Autodesk Inventor part; units mm, degrees
(part 2 of 2)
  line L197 (11.6356, -9.684) -> (11.6356, -8.9363) construction
  line L198 (11.6356, -8.9363) -> (11.5503, -8.9363) construction
  line L199 (11.5503, -8.9363) -> (11.5503, -9.8863) construction
  line L200 (11.5503, -9.8863) -> (11.5697, -9.8863) construction
  line L201 (11.5697, -9.8863) -> (12.1958, -9.1403) construction
  line L202 (12.1958, -9.1403) -> (12.1958, -9.8863) construction
  spline S63 degree 3 poles (12.9637, -8.912) (12.9539, -8.9121) (12.9344, -8.9124) (12.9054, -8.9146) (12.8768, -8.918) (12.8486, -8.9227) (12.8209, -8.9291) (12.7937, -8.9367) (12.7668, -8.9456) (12.7405, -8.9562) (12.7144, -8.9682) (12.6884, -8.9817) (12.6627, -8.9969) (12.6371, -9.014) (12.6116, -9.0325) (12.5866, -9.0531) (12.5613, -9.0749) (12.5451, -9.0905) (12.5369, -9.0985) knots 0 0 0 0 0.061617 0.122179 0.182216 0.241864 0.30096 0.359969 0.419033 0.478069 0.537993 0.59896 0.661321 0.725248 0.79122 0.858746 0.928318 1 1 1 1 construction
  line L203 (12.5369, -9.0985) -> (12.6099, -9.1677) construction
  spline S64 degree 3 poles (12.6099, -9.1677) (12.6232, -9.1553) (12.6493, -9.1307) (12.6919, -9.0988) (12.7363, -9.0715) (12.7824, -9.0493) (12.829, -9.0315) (12.8753, -9.0189) (12.9211, -9.0108) (12.9516, -9.0099) (12.9666, -9.0094) knots 0 0 0 0 0.136144 0.269043 0.398517 0.5271 0.652283 0.77168 0.887495 1 1 1 1 construction
  spline S65 degree 3 poles (12.9666, -9.0094) (12.9758, -9.0095) (12.9942, -9.0097) (13.0215, -9.0126) (13.0485, -9.0167) (13.0752, -9.0227) (13.1016, -9.0302) (13.1276, -9.0397) (13.1533, -9.0507) (13.1784, -9.0634) (13.2028, -9.0774) (13.2258, -9.0929) (13.2476, -9.1094) (13.2678, -9.1273) (13.2865, -9.1465) (13.3041, -9.1666) (13.32, -9.1881) (13.3345, -9.2108) (13.3473, -9.234) (13.3587, -9.2578) (13.3682, -9.2819) (13.3757, -9.3063) (13.3819, -9.331) (13.3863, -9.3561) (13.3888, -9.3815) (13.3892, -9.3986) (13.3894, -9.4071) knots 0 0 0 0 0.042841 0.085571 0.127719 0.170068 0.212787 0.255482 0.298877 0.342861 0.386528 0.429532 0.471886 0.513729 0.555082 0.596535 0.63812 0.679822 0.721331 0.761888 0.802199 0.841806 0.88106 0.920633 0.960101 1 1 1 1 construction
  spline S66 degree 3 poles (13.3894, -9.4071) (13.3892, -9.4159) (13.3888, -9.4334) (13.3862, -9.4595) (13.3813, -9.4852) (13.3748, -9.5107) (13.3667, -9.5358) (13.3565, -9.5606) (13.3445, -9.585) (13.3306, -9.6089) (13.3154, -9.6321) (13.2983, -9.6539) (13.2801, -9.6747) (13.2603, -9.694) (13.2393, -9.7123) (13.2166, -9.7291) (13.1927, -9.7447) (13.1674, -9.7589) (13.1412, -9.7716) (13.1142, -9.7829) (13.0865, -9.7922) (13.0582, -9.7998) (13.0294, -9.806) (12.9998, -9.81) (12.9697, -9.8129) (12.9494, -9.8131) (12.9392, -9.8133) knots 0 0 0 0 0.038994 0.077882 0.116652 0.155416 0.194618 0.234261 0.274547 0.315667 0.35702 0.398083 0.439098 0.479833 0.521274 0.562841 0.605292 0.648409 0.691727 0.735149 0.778369 0.821661 0.865524 0.909731 0.954523 1 1 1 1 construction
  spline S67 degree 3 poles (12.9392, -9.8133) (12.9268, -9.813) (12.9027, -9.8125) (12.8671, -9.8086) (12.833, -9.8024) (12.8003, -9.7934) (12.7691, -9.7819) (12.7393, -9.7681) (12.7111, -9.7514) (12.6843, -9.7325) (12.6597, -9.7114) (12.6375, -9.6887) (12.618, -9.6645) (12.6011, -9.6388) (12.587, -9.6115) (12.5755, -9.5827) (12.5667, -9.5524) (12.5631, -9.5315) (12.5612, -9.5209) knots 0 0 0 0 0.07063 0.138694 0.204918 0.269441 0.332636 0.395302 0.457764 0.520657 0.582852 0.643315 0.70258 0.760908 0.81949 0.878269 0.938491 1 1 1 1 construction
  line L204 (12.5612, -9.5209) -> (12.8779, -9.5209) construction
  line L205 (12.8779, -9.5209) -> (12.8779, -9.4235) construction
  line L206 (12.8779, -9.4235) -> (12.476, -9.4235) construction
  spline S68 degree 3 poles (12.476, -9.4235) (12.4764, -9.4417) (12.4773, -9.4772) (12.4837, -9.5291) (12.494, -9.578) (12.508, -9.6241) (12.5261, -9.6674) (12.5482, -9.7078) (12.5746, -9.7451) (12.6043, -9.7796) (12.6377, -9.8103) (12.6738, -9.8373) (12.7126, -9.8601) (12.7543, -9.8787) (12.7985, -9.8931) (12.8455, -9.9034) (12.8952, -9.9095) (12.9292, -9.9103) (12.9466, -9.9107) knots 0 0 0 0 0.071272 0.139493 0.204635 0.267406 0.328446 0.388397 0.447734 0.507392 0.566768 0.625478 0.684067 0.743248 0.804033 0.866499 0.931723 1 1 1 1 construction
  spline S69 degree 3 poles (12.9466, -9.9107) (12.9573, -9.9105) (12.9785, -9.9102) (13.0097, -9.9081) (13.0401, -9.9047) (13.0696, -9.8997) (13.0983, -9.8935) (13.1262, -9.8856) (13.1533, -9.8765) (13.1796, -9.8661) (13.2049, -9.8541) (13.2293, -9.8407) (13.253, -9.826) (13.2758, -9.8098) (13.2978, -9.7923) (13.3189, -9.7732) (13.3391, -9.7528) (13.3518, -9.7383) (13.3582, -9.731) knots 0 0 0 0 0.069237 0.136557 0.202094 0.266464 0.329769 0.391879 0.453271 0.514115 0.57439 0.634142 0.693923 0.754152 0.81447 0.875661 0.937348 1 1 1 1 construction
  spline S70 degree 3 poles (13.3582, -9.731) (13.3675, -9.7195) (13.3859, -9.6965) (13.4096, -9.6597) (13.4298, -9.6216) (13.4462, -9.5821) (13.459, -9.5412) (13.4681, -9.499) (13.4735, -9.4554) (13.4743, -9.4259) (13.4747, -9.411) knots 0 0 0 0 0.127896 0.253668 0.376738 0.499344 0.621999 0.745699 0.871345 1 1 1 1 construction
  spline S71 degree 3 poles (13.4747, -9.411) (13.4745, -9.3998) (13.4743, -9.3776) (13.4708, -9.3446) (13.4658, -9.3122) (13.4584, -9.2805) (13.4492, -9.2493) (13.4376, -9.2187) (13.4242, -9.1886) (13.4086, -9.1593) (13.3912, -9.1312) (13.3723, -9.1044) (13.3516, -9.0793) (13.3296, -9.0556) (13.3059, -9.0337) (13.2807, -9.0133) (13.2541, -8.9944) (13.2258, -8.9773) (13.1965, -8.9619) (13.1661, -8.9485) (13.1346, -8.9373) (13.1023, -8.9279) (13.0689, -8.9209) (13.0348, -8.9159) (12.9996, -8.9124) (12.9758, -8.9121) (12.9637, -8.912) knots 0 0 0 0 0.042039 0.083544 0.124643 0.165303 0.206171 0.246971 0.288329 0.329987 0.371797 0.412738 0.453459 0.494001 0.534381 0.574952 0.615892 0.65725 0.699007 0.740486 0.782325 0.824567 0.867041 0.9105 0.954619 1 1 1 1 construction
  line L207 (47.1288, -8.7194) -> (47.1288, -7.7194) construction
  line L208 (47.1288, -7.7194) -> (46.9026, -7.7194) construction
  spline S72 degree 3 poles (46.9026, -7.7194) (46.885, -7.7196) (46.8509, -7.7198) (46.8015, -7.7225) (46.7556, -7.7266) (46.7131, -7.7323) (46.6742, -7.7398) (46.6388, -7.7492) (46.6068, -7.7601) (46.578, -7.7729) (46.5517, -7.7879) (46.5267, -7.8045) (46.5031, -7.8234) (46.4805, -7.8443) (46.4593, -7.8675) (46.439, -7.8927) (46.4202, -7.9201) (46.4024, -7.9492) (46.3862, -7.9801) (46.3721, -8.0125) (46.3603, -8.0462) (46.3507, -8.0812) (46.3431, -8.1175) (46.3377, -8.155) (46.3344, -8.1938) (46.3341, -8.2201) (46.3339, -8.2335) knots 0 0 0 0 0.060148 0.116267 0.168654 0.217399 0.262434 0.303933 0.34226 0.377441 0.411406 0.445398 0.479766 0.514584 0.550214 0.587001 0.624663 0.663615 0.703456 0.74345 0.784013 0.825133 0.867265 0.910306 0.954424 1 1 1 1 construction
  spline S73 degree 3 poles (46.3339, -8.2335) (46.3344, -8.2523) (46.3353, -8.2894) (46.3427, -8.3439) (46.3546, -8.3961) (46.3715, -8.4457) (46.3923, -8.4921) (46.4172, -8.5346) (46.4459, -8.573) (46.4778, -8.607) (46.5125, -8.6363) (46.5485, -8.6613) (46.5861, -8.6811) (46.6194, -8.6936) (46.6482, -8.7014) (46.6734, -8.706) (46.7022, -8.7102) (46.7346, -8.7135) (46.7706, -8.7164) (46.8103, -8.7179) (46.8536, -8.7193) (46.8836, -8.7194) (46.8992, -8.7194) knots 0 0 0 0 0.065773 0.129478 0.19143 0.252446 0.311787 0.368818 0.424092 0.478492 0.531394 0.582004 0.631201 0.679503 0.705561 0.735222 0.769132 0.806858 0.84893 0.895117 0.94547 1 1 1 1 construction
  line L209 (46.8992, -8.7194) -> (47.1288, -8.7194) construction
  line L210 (47.8467, -8.7194) -> (47.8467, -7.7194) construction
  line L211 (47.8467, -7.7194) -> (47.3083, -7.7194) construction
  line L212 (47.3083, -7.7194) -> (47.3083, -7.8989) construction
  line L213 (47.3083, -7.8989) -> (47.6673, -7.8989) construction
  line L214 (47.6673, -7.8989) -> (47.6673, -8.0912) construction
  line L215 (47.6673, -8.0912) -> (47.3083, -8.0912) construction
  line L216 (47.3083, -8.0912) -> (47.3083, -8.2707) construction
  line L217 (47.3083, -8.2707) -> (47.6673, -8.2707) construction
  line L218 (47.6673, -8.2707) -> (47.6673, -8.54) construction
  line L219 (47.6673, -8.54) -> (47.3083, -8.54) construction
  line L220 (47.3083, -8.54) -> (47.3083, -8.7194) construction
  line L221 (47.3083, -8.7194) -> (47.8467, -8.7194) construction
  line L222 (48.4621, -8.7194) -> (48.4621, -7.7194) construction
  line L223 (48.4621, -7.7194) -> (48.2826, -7.7194) construction
  line L224 (48.2826, -7.7194) -> (48.2826, -8.54) construction
  line L225 (48.2826, -8.54) -> (48.0006, -8.54) construction
  line L226 (48.0006, -8.54) -> (48.0006, -8.7194) construction
  line L227 (48.0006, -8.7194) -> (48.4621, -8.7194) construction
  circle A18 centre (48.35, -12.79) radius 0.75 construction
  circle A19 centre (48.35, -10.25) radius 0.75 construction
  circle A20 centre (9.37, -17.12) radius 0.75 construction
  circle A21 centre (9.37, -14.58) radius 0.75 construction
  circle A22 centre (9.37, -12.04) radius 0.75 construction
  circle A23 centre (9.37, -9.5) radius 0.75 construction
  line L228 (25.55, -16.65) -> (24.65, -16.65) construction
  line L229 (25.55, -15.85) -> (25.55, -16.65) construction
  line L230 (24.65, -15.85) -> (25.55, -15.85) construction
  line L231 (24.65, -16.65) -> (24.65, -15.85) construction
  line L232 (25.55, -15.35) -> (24.65, -15.35) construction
  line L233 (25.55, -14.55) -> (25.55, -15.35) construction
  line L234 (24.65, -14.55) -> (25.55, -14.55) construction
  line L235 (24.65, -15.35) -> (24.65, -14.55) construction
  line L236 (25.55, -14.05) -> (24.65, -14.05) construction
  line L237 (25.55, -13.25) -> (25.55, -14.05) construction
  line L238 (24.65, -13.25) -> (25.55, -13.25) construction
  line L239 (24.65, -14.05) -> (24.65, -13.25) construction
  line L240 (25.55, -12.75) -> (24.65, -12.75) construction
  line L241 (25.55, -11.95) -> (25.55, -12.75) construction
  line L242 (24.65, -11.95) -> (25.55, -11.95) construction
  line L243 (24.65, -12.75) -> (24.65, -11.95) construction
  line L244 (25.55, -11.45) -> (24.65, -11.45) construction
  line L245 (25.55, -10.65) -> (25.55, -11.45) construction
  line L246 (24.65, -10.65) -> (25.55, -10.65) construction
  line L247 (24.65, -11.45) -> (24.65, -10.65) construction
  line L248 (25.55, -10.15) -> (24.65, -10.15) construction
  line L249 (25.55, -9.35) -> (25.55, -10.15) construction
  line L250 (24.65, -9.35) -> (25.55, -9.35) construction
  line L251 (24.65, -10.15) -> (24.65, -9.35) construction
  line L252 (25.55, -8.85) -> (24.65, -8.85) construction
  line L253 (25.55, -8.05) -> (25.55, -8.85) construction
  line L254 (24.65, -8.05) -> (25.55, -8.05) construction
  line L255 (24.65, -8.85) -> (24.65, -8.05) construction
  line L256 (25.55, -17.15) -> (25.55, -17.95) construction
  line L257 (24.65, -17.15) -> (25.55, -17.15) construction
  line L258 (24.65, -17.95) -> (24.65, -17.15) construction
  line L259 (25.55, -17.95) -> (24.65, -17.95) construction
  line L260 (26.5, -7.75) -> (33.8, -7.75) construction
  line L261 (26.5, -18.25) -> (26.5, -7.75) construction
  line L262 (33.8, -18.25) -> (26.5, -18.25) construction
  line L263 (33.8, -7.75) -> (33.8, -18.25) construction
  line L264 (34.75, -8.05) -> (35.65, -8.05) construction
  line L265 (34.75, -8.05) -> (34.75, -8.85) construction
  line L266 (35.65, -8.85) -> (34.75, -8.85) construction
  line L267 (35.65, -8.05) -> (35.65, -8.85) construction
  line L268 (34.75, -9.35) -> (35.65, -9.35) construction
  line L269 (34.75, -9.35) -> (34.75, -10.15) construction
  line L270 (35.65, -10.15) -> (34.75, -10.15) construction
  line L271 (35.65, -9.35) -> (35.65, -10.15) construction
  line L272 (34.75, -10.65) -> (35.65, -10.65) construction
  line L273 (34.75, -10.65) -> (34.75, -11.45) construction
  line L274 (35.65, -11.45) -> (34.75, -11.45) construction
  line L275 (35.65, -10.65) -> (35.65, -11.45) construction
  line L276 (34.75, -11.95) -> (35.65, -11.95) construction
  line L277 (34.75, -11.95) -> (34.75, -12.75) construction
  line L278 (35.65, -12.75) -> (34.75, -12.75) construction
  line L279 (35.65, -11.95) -> (35.65, -12.75) construction
  line L280 (34.75, -13.25) -> (35.65, -13.25) construction
  line L281 (34.75, -13.25) -> (34.75, -14.05) construction
  line L282 (35.65, -14.05) -> (34.75, -14.05) construction
  line L283 (35.65, -13.25) -> (35.65, -14.05) construction
  line L284 (34.75, -14.55) -> (35.65, -14.55) construction
  line L285 (34.75, -14.55) -> (34.75, -15.35) construction
  line L286 (35.65, -15.35) -> (34.75, -15.35) construction
  line L287 (35.65, -14.55) -> (35.65, -15.35) construction
  line L288 (34.75, -15.85) -> (35.65, -15.85) construction
  line L289 (34.75, -15.85) -> (34.75, -16.65) construction
  line L290 (35.65, -16.65) -> (34.75, -16.65) construction
  line L291 (35.65, -15.85) -> (35.65, -16.65) construction
  line L292 (34.75, -17.15) -> (35.65, -17.15) construction
  line L293 (34.75, -17.15) -> (34.75, -17.95) construction
  line L294 (35.65, -17.95) -> (34.75, -17.95) construction
  line L295 (35.65, -17.15) -> (35.65, -17.95) construction
  circle A24 centre (45.56, -5.5) radius 0.75 construction
  circle A25 centre (48.1, -5.5) radius 0.75 construction
  line L296 (50.7939, -3) -> (5.9071, -3) construction
  line L297 (5.9071, -3) -> (5.9071, -23.644) construction
  line L298 (5.9071, -23.644) -> (50.7939, -23.644) construction
  line L299 (50.7939, -23.644) -> (50.7939, -3) construction
  line L300 (50.7939, -23.644) -> (5.9071, -23.644)
  line L301 (5.9071, -23.644) -> (5.9071, -3)
  line L302 (5.9071, -3) -> (50.7939, -3)
  line L303 (50.7939, -3) -> (50.7939, -23.644)
  line L304 (93.3881, -56.8601) -> (4, -56.8601)
  line L305 (4, -56.8601) -> (4, -8.85)
  line L306 (4, -8.85) -> (93.3881, -8.85)
  line L307 (93.3881, -8.85) -> (93.3881, -56.8601)
  point P0 (0, -3)
  constraints: 24 end point, 6 parallel, 3 horizontal, 3 perpendicular
extrude "Extrusion5" cut sketch "Sketch5" against normal blind 3
sketch "Sketch6" plane through (103, 6.6, 3) normal (1, 0, 0) x (0, 0, -1)
  line L0 (32.7723, 17.3458) -> (40.0033, 0.6221) projected
  arc A0 (33.8143, 19.9753) -> (32.7723, 17.3458) centre (34.6081, 18.1395) ccw projected
  line L1 (49.8404, 26.9047) -> (33.8143, 19.9753) projected
  arc A1 (52.4699, 25.8626) -> (49.8404, 26.9047) centre (50.6341, 25.0689) ccw projected
  line L2 (59.7009, 9.139) -> (52.4699, 25.8626) projected
  arc A2 (58.6589, 6.5095) -> (59.7009, 9.139) centre (57.8651, 8.3452) ccw projected
  line L3 (42.6328, -0.4199) -> (58.6589, 6.5095) projected
  arc A3 (40.0033, 0.6221) -> (42.6328, -0.4199) centre (41.8391, 1.4159) ccw projected
  arc A4 (58.778, 6.2341) -> (59.9763, 9.2581) centre (57.8651, 8.3452) ccw
  line L4 (59.9763, 9.2581) -> (52.7452, 25.9817)
  arc A5 (52.7452, 25.9817) -> (49.7213, 27.18) centre (50.6341, 25.0689) ccw
  line L5 (49.7213, 27.18) -> (33.6952, 20.2506)
  arc A6 (33.6952, 20.2506) -> (32.4969, 17.2267) centre (34.6081, 18.1395) ccw
  line L6 (32.4969, 17.2267) -> (39.728, 0.503)
  arc A7 (39.728, 0.503) -> (42.7519, -0.6953) centre (41.8391, 1.4159) ccw
  line L7 (42.7519, -0.6953) -> (58.778, 6.2341)
  point P0 (3, -6.6)
  dimension "d16" = 0.3
  constraints: 8 end point, 8 point on circle, 4 centre point, 7 other
  measures "d16" distance between parallel lines of L3 L7
extrude "Extrusion6" cut sketch "Sketch6" against normal through all contours A0 L1 A1 L2 A2 L3 A3 L0 | L7 A7 L6 A6 L5 A5 L4 A4
sketch "Sketch7" plane through (-2, 6.6, 0) normal (1, 0, 0) x (0, 0, -1)
  arc A0 (36.728, 0.503) -> (37.0265, 0) centre (38.8391, 1.4159) ccw projected
  line L0 (36.728, 0.503) -> (29.4969, 17.2267) projected
  arc A1 (30.6952, 20.2506) -> (29.4969, 17.2267) centre (31.6081, 18.1395) ccw projected
  line L1 (30.6952, 20.2506) -> (46.7213, 27.18) projected
  arc A2 (49.7452, 25.9817) -> (46.7213, 27.18) centre (47.6341, 25.0689) ccw projected
  line L2 (49.7452, 25.9817) -> (56.9763, 9.2581) projected
  arc A3 (55.778, 6.2341) -> (56.9763, 9.2581) centre (54.8651, 8.3452) ccw projected
  line L3 (55.778, 6.2341) -> (41.3598, 0) projected
  line L4 (41.3598, 0) -> (60, 0) projected
  line L5 (60, 0) -> (60, 4.0286) projected
  line L6 (60, 4.0286) -> (27.1513, 80) projected
  line L7 (-3, 80) -> (27.1513, 80) projected
  line L8 (-3, 0) -> (-3, 80) projected
  line L9 (-3, 0) -> (37.0265, 0) projected
  circle A4 centre (17.557, 24.8509) radius 11.8979 projected
  line L10 (45.542, 26.6701) -> (30.6952, 20.2506)
  line L11 (30.6952, 20.2506) -> (29.5936, 22.7985)
  line L12 (29.5936, 22.7985) -> (44.4403, 29.218)
  line L13 (44.4403, 29.218) -> (45.542, 26.6701)
  line L14 (29.4969, 17.2267) -> (37.0265, 0)
  line L15 (37.0265, 0) -> (33.9632, -1.339)
  line L16 (33.9632, -1.339) -> (26.4336, 15.8878)
  line L17 (26.4336, 15.8878) -> (29.4969, 17.2267)
  line L18 (54.8651, 5.8395) -> (41.3598, 0)
  line L19 (57.4122, -0.0512) -> (54.8651, 5.8395)
  line L20 (29.5936, 22.7985) -> (29.2312, 22.5542)
  line L21 (26.4336, 15.8878) -> (26.1097, 16.5797)
  line L22 (44.4403, 29.218) -> (48.3733, 30.9185)
  line L23 (33.9632, -1.339) -> (35.3257, -4.4564)
  line L24 (35.3257, -4.4564) -> (60, -4.4564)
  line L25 (41.3598, 0) -> (60, 0) projected
  line L26 (60, -4.4564) -> (60, 4.0286)
  point P0 (0, -6.6)
  constraints: 32 end point, 5 parallel, 5 point on line, 3 perpendicular, 2 point on circle, 1 collinear, 2 other
extrude "Extrusion7" add sketch "Sketch7" along normal blind 15 contours L0 L14 A0 | A0 L9 L16 L17 L0 | L15 L16 L9 | L14 A1 L1 A2 L2 A3 L3 L4 L26 L24 L23 L15 | L17 L21 A4 L20 L11 A1 | L11 L12 L13 L1 | L13 L22 L6 L5 L4 L19 L3 A3 L2 A2 L1 | A4 | L4 L3 L19
sketch "Sketch8" plane through (-5, 6.6, 3) normal (-1, 0, 0) x (0, 0, 1)
  line L0 (-42.7519, -0.6953) -> (-58.778, 6.2341) projected
  arc A0 (-42.7519, -0.6953) -> (-39.728, 0.503) centre (-41.8391, 1.4159) ccw projected
  line L1 (-39.728, 0.503) -> (-32.4969, 17.2267) projected
  arc A1 (-32.4969, 17.2267) -> (-33.6952, 20.2506) centre (-34.6081, 18.1395) ccw projected
  line L2 (-33.6952, 20.2506) -> (-49.7213, 27.18) projected
  arc A2 (-49.7213, 27.18) -> (-52.7452, 25.9817) centre (-50.6341, 25.0689) ccw projected
  line L3 (-52.7452, 25.9817) -> (-59.9763, 9.2581) projected
  arc A3 (-59.9763, 9.2581) -> (-58.778, 6.2341) centre (-57.8651, 8.3452) ccw projected
  circle A4 centre (-20.557, 24.8509) radius 10.6399 projected
  circle A5 centre (-20.557, 24.8509) radius 11.9384
  point P0 (-3, -6.6)
  constraints: 1 centre point
extrude "Extrusion8" cut sketch "Sketch8" against normal through all contours L0 A3 L3 A2 L2 A1 L1 A0 | A4 | A5
sketch "Sketch9" plane through (100, 6.6, 0) normal (-1, 0, 0) x (0, 0, 1)
  arc A0 (-29.2786, 22.5862) -> (-26.1281, 16.5405) centre (-17.557, 24.8509) ccw projected
  line L0 (-53.8601, -2) -> (-53.8601, -4.4564) projected
  line L1 (-60, -2) -> (-53.8601, -2) projected
  line L2 (-60, -2) -> (-60, 4.0286) projected
  line L3 (-60, 4.0286) -> (-48.3733, 30.9185) projected
  line L4 (-48.3733, 30.9185) -> (-29.5936, 22.7985) projected
  line L5 (-29.5936, 22.7985) -> (-29.2786, 22.5862) projected
  line L6 (-26.1281, 16.5405) -> (-26.4336, 15.8878) projected
  line L7 (-26.4336, 15.8878) -> (-35.3257, -4.4564) projected
  line L8 (-35.3257, -4.4564) -> (-53.8601, -4.4564) projected
  line L9 (-41.5802, 6.1987) -> (-40.8052, 7.9911) projected
  line L10 (-40.8052, 7.9911) -> (-48.7279, 11.4167) projected
  line L11 (-48.7279, 11.4167) -> (-49.5029, 9.6243) projected
  line L12 (-49.5029, 9.6243) -> (-41.5802, 6.1987) projected
  line L13 (-36.158, 12.8961) -> (-34.2689, 17.2651) projected
  line L14 (-34.2689, 17.2651) -> (-46.4486, 22.5313) projected
  line L15 (-46.4486, 22.5313) -> (-48.3377, 18.1624) projected
  line L16 (-48.3377, 18.1624) -> (-36.158, 12.8961) projected
  line L17 (-29.7723, 17.3458) -> (-37.0033, 0.6221) projected
  arc A1 (-39.6328, -0.4199) -> (-37.0033, 0.6221) centre (-38.8391, 1.4159) ccw projected
  line L18 (-39.6328, -0.4199) -> (-55.6589, 6.5095) projected
  arc A2 (-56.7009, 9.139) -> (-55.6589, 6.5095) centre (-54.8651, 8.3452) ccw projected
  line L19 (-56.7009, 9.139) -> (-49.4699, 25.8626) projected
  arc A3 (-46.8404, 26.9047) -> (-49.4699, 25.8626) centre (-47.6341, 25.0689) ccw projected
  line L20 (-46.8404, 26.9047) -> (-30.8143, 19.9753) projected
  arc A4 (-29.7723, 17.3458) -> (-30.8143, 19.9753) centre (-31.6081, 18.1395) ccw projected
  line L21 (-36.8772, 0.5676) -> (-29.6462, 17.2912)
  arc A5 (-29.6462, 17.2912) -> (-30.7598, 20.1014) centre (-31.6081, 18.1395) ccw
  line L22 (-30.7598, 20.1014) -> (-46.7859, 27.0308)
  arc A6 (-46.7859, 27.0308) -> (-49.596, 25.9172) centre (-47.6341, 25.0689) ccw
  line L23 (-49.596, 25.9172) -> (-56.827, 9.1935)
  arc A7 (-56.827, 9.1935) -> (-55.7134, 6.3834) centre (-54.8651, 8.3452) ccw
  line L24 (-55.7134, 6.3834) -> (-39.6873, -0.546)
  arc A8 (-39.6873, -0.546) -> (-36.8772, 0.5676) centre (-38.8391, 1.4159) ccw
  point P0 (0, -6.6)
  constraints: 8 end point, 8 point on circle, 4 centre point, 7 other
extrude "Extrusion9" add sketch "Sketch9" along normal blind 10 contours A0 L6 L7 L8 L0 L1 L2 L3 L4 L5 | A8 L24 A7 L23 A6 L22 A5 L21
sketch "Sketch10" plane through (0, 0, 0) normal (0, 0, -1) x (-1, 0, 0)
  line L0 (5, 10.6286) -> (-13, 10.6286) projected
  line L1 (5, 86.6) -> (5, 10.6286) projected
  arc A0 (5, 86.6) -> (0, 91.6) centre (0, 86.6) ccw projected
  line L2 (-98, 91.6) -> (0, 91.6) projected
  arc A1 (-98, 91.6) -> (-103, 86.6) centre (-98, 86.6) ccw projected
  line L3 (-103, 10.6286) -> (-103, 86.6) projected
  line L4 (-90, 10.6286) -> (-103, 10.6286) projected
  line L5 (-90, 37.5185) -> (-90, 10.6286) projected
  line L6 (-100, 37.5185) -> (-90, 37.5185) projected
  line L7 (-100, 86.6) -> (-100, 37.5185) projected
  arc A2 (-98, 88.6) -> (-100, 86.6) centre (-98, 86.6) ccw projected
  line L8 (0, 88.6) -> (-98, 88.6) projected
  arc A3 (2, 86.6) -> (0, 88.6) centre (0, 86.6) ccw projected
  line L9 (2, 37.5185) -> (2, 86.6) projected
  line L10 (2, 37.5185) -> (-13, 37.5185) projected
  line L11 (-13, 10.6286) -> (-13, 37.5185) projected
  circle A4 centre (0, 86.6) radius 2 construction
  circle A5 centre (0, 86.6) radius 5
  circle A6 centre (-98, 86.6) radius 2 construction
  circle A7 centre (-98, 86.6) radius 5
  circle A8 centre (0, 86.6) radius 1.45
  circle A9 centre (-98, 86.6) radius 1.45
  point P0 (0, 0)
  dimension "d27" = 2.9
  dimension "d28" = 2.9
  constraints: 6 centre point, 6 coincident, 3 concentric
  measures "d27" diameter of A8
  measures "d28" diameter of A9
extrude "Extrusion10" add sketch "Sketch10" along normal up to surface contours A5 L9 A3 L8 A0 | A5 L8 A3 L9 | A7 L8 A2 L7 A1 | A7 L7 A2 L8 surface through (-5, 93.7327, -24.0673) normal (0, -0.3968725, 0.9178738)
sketch "Sketch11" plane through (98, 1.6, -60) normal (0, 0, -1) x (-1, 0, 0)
  line L0 (8, 9.0286) -> (-5, 9.0286) projected
  line L1 (-5, 5) -> (-5, 9.0286) projected
  arc A0 (-5, 5) -> (0, 0) centre (0, 5) ccw projected
  line L2 (98, 0) -> (0, 0) projected
  arc A1 (98, 0) -> (103, 5) centre (98, 5) ccw projected
  line L3 (103, 9.0286) -> (103, 5) projected
  line L4 (103, 9.0286) -> (85, 9.0286) projected
  line L5 (85, 3) -> (85, 9.0286) projected
  line L6 (8, 3) -> (85, 3) projected
  line L7 (8, 9.0286) -> (8, 3) projected
  circle A2 centre (98, 5) radius 1.45
  circle A3 centre (0, 5) radius 1.45
  point P0 (98, -1.6)
  dimension "d29" = 2.9
  dimension "d30" = 2.9
  constraints: 2 centre point, 2 coincident
  measures "d29" diameter of A2
  measures "d30" diameter of A3
extrude "Extrusion11" cut sketch "Sketch11" against normal blind 20 contours A2 | A3
sketch "Sketch12" plane through (4, 2.1436, -53.8601) normal (0, -1, 0) x (1, 0, 0)
  circle A0 centre (-1.5, -3.6399) radius 1.5 projected
  circle A1 centre (91.5, -3.6399) radius 1.5 projected
  point P0 (-4, 53.8601)
extrude "Extrusion12" cut sketch "Sketch12" against normal blind 20
sketch "Sketch13" plane through (103, 6.6, 3) normal (1, 0, 0) x (0, 0, -1)
  circle A0 centre (20.557, 24.8509) radius 11.9384 projected
  arc A1 (39.728, 0.503) -> (40.0265, 0) centre (41.8391, 1.4159) ccw projected
  line L0 (39.728, 0.503) -> (32.4969, 17.2267) projected
  arc A2 (33.6952, 20.2506) -> (32.4969, 17.2267) centre (34.6081, 18.1395) ccw projected
  line L1 (33.6952, 20.2506) -> (49.7213, 27.18) projected
  arc A3 (52.7452, 25.9817) -> (49.7213, 27.18) centre (50.6341, 25.0689) ccw projected
  line L2 (52.7452, 25.9817) -> (59.9763, 9.2581) projected
  arc A4 (58.778, 6.2341) -> (59.9763, 9.2581) centre (57.8651, 8.3452) ccw projected
  line L3 (58.778, 6.2341) -> (44.3598, 0) projected
  line L4 (44.3598, 0) -> (63, 0) projected
  line L5 (63, 0) -> (63, 4.0286) projected
  line L6 (63, 4.0286) -> (30.1513, 80) projected
  line L7 (0, 80) -> (30.1513, 80) projected
  line L8 (0, 0) -> (0, 80) projected
  line L9 (0, 0) -> (40.0265, 0) projected
  line L10 (3, 75.4174) -> (32.1327, 75.4174) projected
  line L11 (9.8433, 61.5372) -> (8.9292, 61.5372)
  line L12 (5.9292, 64.5372) -> (5.9292, 72.4174)
  line L13 (8.9292, 75.4174) -> (9.8433, 75.4174)
  line L14 (12.8433, 72.4174) -> (12.8433, 64.5372)
  arc A5 (9.8433, 61.5372) -> (12.8433, 64.5372) centre (9.8433, 64.5372) ccw
  arc A6 (5.9292, 64.5372) -> (8.9292, 61.5372) centre (8.9292, 64.5372) ccw
  arc A7 (8.9292, 75.4174) -> (5.9292, 72.4174) centre (8.9292, 72.4174) ccw
  arc A8 (12.8433, 72.4174) -> (9.8433, 75.4174) centre (9.8433, 72.4174) ccw
  point P0 (3, -6.6)
  point P1 (5.9292, 75.4174)
  dimension "d35" = 3
  constraints: 8 end point, 8 point on circle, 8 tangent, 4 centre point, 3 equal radius, 3 point on line, 2 parallel, 1 horizontal, 1 perpendicular
  measures "d35" radius of A5
extrude "Extrusion13" cut sketch "Sketch13" against normal through all contours L10 A8 L14 A5 L11 A6 L12 A7
sketch "Sketch14" plane through (4.5826, 88.6, 0) normal (0, -1, 0) x (1, 0, 0)
  circle A0 centre (10.2397, -17.557) radius 7.21 projected
  line L0 (-9.5826, 3) -> (-4.5826, 3) projected
  line L1 (-4.5826, 3) -> (93.4174, 3) projected
  line L2 (93.4174, 3) -> (98.4174, 3) projected
  line L3 (98.4174, 3) -> (93.4174, 3) projected
  line L4 (93.4174, 3) -> (-4.5826, 3) projected
  line L5 (-4.5826, 3) -> (-9.5826, 3) projected
  line L6 (0, 0) -> (88.8348, 0) projected
  line L7 (0.4174, 0) -> (0.4174, -27.1513) projected
  line L8 (-2.5826, -5.9292) -> (-2.5826, -6.8433) projected
  line L9 (-6.5826, -29.1327) -> (-6.5826, -6.8433) projected
  ellipse E0 centre (-4.5826, -27.1513) end of major axis (-9.5826, -27.1513) minor radius 2.1619 (-6.5826, -29.1327) -> (0, -26.2865) ccw projected
  line L10 (0, 0) -> (0, -26.2865) projected
  line L11 (-6.5826, 0) -> (0, 0) projected
  line L12 (-6.5826, -5.9292) -> (-6.5826, 0) projected
  circle A1 centre (10.2397, -17.557) radius 7.4647
  line L13 (0, -26.2865) -> (22, -26.2865)
  line L14 (0, -26.2865) -> (88.8348, -26.2865) projected
  line L15 (22, -26.2865) -> (22, 0)
  line L16 (22, 0) -> (0, 0)
  line L17 (0, 0) -> (0, -26.2865)
  line L18 (17.7044, -17.557) -> (22, -17.557)
  line L19 (17.7044, -17.557) -> (22, -17.557) construction
  line L20 (2.7751, -17.557) -> (0, -17.557)
  line L21 (0, 0) -> (0, -26.2865) projected
  line L22 (2.7751, -17.557) -> (5.5502, -17.557) construction
  point P0 (-4.5826, 0)
  dimension "d38" = 22
  dimension "d39" = 90
  dimension "d40" = 0
  dimension "d41" = 180
  constraints: 16 end point, 4 point on line, 3 collinear, 2 horizontal, 2 horizontal alignment, 2 point on circle, 1 centre point, 1 perpendicular, 1 other
  measures "d38" distance of L10.end L13.end
  measures "d39" angle of L15 L13
  measures "d40" distance between parallel lines of L18 L19
  measures "d41" angle of L20 L22
extrude "Extrusion14" add sketch "Sketch14" along normal blind 11 contours L6 L7 L20 L10 | L6 L15 L18 A1 L20 L7
chamfer "Chamfer1" distance 2 angle 45 1 edges at (14.8223, 77.6, -10.0924)
body "Solid1"
